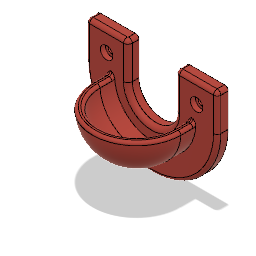
BallCatcher (Autodesk Fusion 360 design; units mm, degrees)
Autodesk Fusion 360 part; units mm, degrees
sphere "SpherePrimitive1" add diameter 60 placed x (1, 0, 0) y (0, 0, -1) z (0, 1, 0) at (0, 0, 0) makes body 1
shell "Shell1" thickness 5 removed faces 0 bodies 1
split "Split1" by plane through (0, 0, 0) normal (0, 0, 1) bodies 1 makes body 2 at (28.4422, -6.3836, 7.0914)
split "Split2" by plane through (0, 0, 0) normal (0, 1, 0) bodies 2 makes body 3 at (-14.8717, 3.9158, 25.7585)
extrude "Extrude1" add 1 faces at (-2.6091, -28.1467, 0) along direction (0, 0, -1) blind 10 on bodies 2 bodies 2
sketch "Sketch2" plane through (0, 0, -10) normal (0, 0, -1) x (-1, 0, 0)
  line L0 (-25, 0) -> (-30, 0)
  arc A0 (-30, 0) -> (30, 0) centre (0, 0) ccw
  line L1 (30, 0) -> (25, 0)
  arc A1 (-25, 0) -> (25, 0) centre (0, 0) ccw
  line L2 (-25, 0) -> (25, 0)
  line L3 (0, 0) -> (48, 0)
  line L4 (0, 0) -> (-53, 0)
  arc A2 (-10.5, 0) -> (10.5, 0) centre (0, 0) ccw
  arc A3 (25, 14.5) -> (10.5, 0) centre (25, 0) ccw
  line L5 (42.0714, 14.5) -> (25, 14.5)
  arc A4 (-42.0714, 14.5) -> (42.0714, 14.5) centre (0, 0) ccw
  line L6 (-25, 14.5) -> (-42.0714, 14.5)
  arc A5 (-10.5, 0) -> (-25, 14.5) centre (-25, 0) ccw
  circle A6 centre (0, 0) radius 16
  dimension "d6" = 14.5
  dimension "d11" = 32
  constraint coincident A0.centre A1.centre
  constraint parallel L2 L3
  constraint parallel L2 L4
  measures "d11" diameter of A6
extrude "Extrude2" add sketch "Sketch2" along normal blind 8 contours L0 A0 L1 A1 L3 L4 | A1 L2 L3 L4 A6 | A0 L3 L4 A4 bodies 2
fillet "Fillet1" radius 3 1 edges at (0, -16, -10) on bodies 2
sketch "Sketch4" plane through (0, 0, 0) normal (0, 1, 0) x (-1, 0, 0)
  arc A0 (19, -10) -> (16, -13) centre (19, -13) ccw
  line L0 (16, -13) -> (16, -18)
  line L1 (16, -18) -> (44.5, -18)
  line L2 (44.5, -18) -> (44.5, -10)
  line L3 (44.5, -10) -> (30, -10)
  line L4 (30, -10) -> (30, 0)
  arc A1 (30, 0) -> (-30, 0) centre (0, 0) ccw
  line L5 (-30, 0) -> (-30, -10)
  line L6 (-30, -10) -> (-44.5, -10)
  line L7 (-44.5, -10) -> (-44.5, -18)
  line L8 (-44.5, -18) -> (-16, -18)
  line L9 (-16, -18) -> (-16, -13)
  arc A2 (-16, -13) -> (-19, -10) centre (-19, -13) ccw
  line L10 (-19, -10) -> (-25, -10)
  line L11 (-25, -10) -> (-25, 0)
  arc A3 (25, 0) -> (-25, 0) centre (0, 0) ccw
  line L12 (25, 0) -> (25, -10)
  line L13 (25, -10) -> (19, -10)
  line L14 (30, -10) -> (25, -10)
  line L15 (-25, -10) -> (-30, -10)
  constraint coincident L3.end L4.start
  constraint coincident L12.end L13.start
  constraint coincident L10.end L11.start
  constraint coincident L5.end L6.start
extrude "Extrude3" add sketch "Sketch4" along normal blind 25 contours A0 L0 L1 L2 L3 L13 L14 | L6 L7 L8 L9 A2 L10 L15 bodies 2
fillet "Fillet2" radius 1.903 1 faces at (26.6667, 0, -6.6667) on bodies 2
fillet "Fillet5" radius 2.5 11 edges at (44.5, 12.5, -10) (0, -44.5, -10) (-44.5, 12.5, -10) (-44.5, 25, -14) (-31.75, 25, -10) (-16.8787, 25, -10.8787) (-16, 25, -15.5) (16, 25, -15.5) (16.8787, 25, -10.8787) (31.75, 25, -10) (44.5, 25, -14) on bodies 2
sketch "Sketch3" plane through (0, 0, -10) normal (0, 0, 1) x (1, 0, 0)
  line L0 (26.8356, 1.903) -> (28.0325, 1.903)
  arc A0 (-29.9631, -1.4874) -> (29.9631, -1.4874) centre (0, 0) ccw
  line L1 (0, -43) -> (0, -30)
  line L2 (0, 0) -> (43, 0) construction
  line L3 (0, 0) -> (43, 0) construction
  arc A1 (-24.9665, -1.2946) -> (24.9665, -1.2946) centre (0, 0) ccw
  spline S0 degree 3 poles (24.9665, -1.2946) (24.9803, -1.0285) (25.038, -0.6917) (25.5642, 0.5413) (26.222, 1.1928) (26.8322, 1.899) (26.8339, 1.901) (26.8356, 1.903) knots 0 0 0 0 0.079915 0.079915 0.246548 0.246548 0.247022 0.247022 0.247022 0.247022
  spline S1 degree 3 poles (28.0325, 1.903) (28.0347, 1.901) (28.037, 1.899) (28.4413, 1.5442) (28.8666, 1.144) (29.4212, 0.3929) (29.6707, 0) (29.9285, -0.8103) (29.9799, -1.1484) (29.9631, -1.4874) knots -0.000904 -0.000904 -0.000904 -0.000904 0 0 0.160455 0.160455 0.251665 0.251665 0.312705 0.312705 0.312705 0.312705
  spline S2 degree 3 poles (-29.9631, -1.4874) (-29.9799, -1.1484) (-29.9285, -0.8103) (-29.6707, 0) (-29.4212, 0.3929) (-28.8666, 1.144) (-28.4413, 1.5442) (-28.037, 1.899) (-28.0347, 1.901) (-28.0325, 1.903) knots 0 0 0 0 0.101851 0.101851 0.254043 0.254043 0.521775 0.521775 0.523283 0.523283 0.523283 0.523283
  line L4 (-28.0325, 1.903) -> (-26.8356, 1.903)
  spline S3 degree 3 poles (-26.8356, 1.903) (-26.8339, 1.901) (-26.8322, 1.899) (-26.222, 1.1928) (-25.5642, 0.5413) (-25.038, -0.6917) (-24.9803, -1.0285) (-24.9665, -1.2946) knots -0.000794 -0.000794 -0.000794 -0.000794 0 0 0.279172 0.279172 0.41306 0.41306 0.41306 0.41306
  line L5 (-19, 0) -> (-19, 22.5)
  line L6 (19, 22.5) -> (19, 0)
  arc A2 (-19, 0) -> (19, 0) centre (0, 0) ccw
  line L7 (-42.0005, -0.0495) -> (-19, 22.5)
  line L8 (19, 22.5) -> (42.0005, -0.0495)
  line L9 (-19, 22.5) -> (-42, 22.5)
  line L10 (-42, 22.5) -> (-42, 0)
  arc A3 (-42, 0) -> (42, 0) centre (0, 0) ccw
  line L11 (42, 0) -> (42, 22.5)
  line L12 (42, 22.5) -> (19, 22.5)
  point P0 (-30.5002, 11.2252)
  point P1 (30.5002, 11.2252)
  constraint midpoint A0 L1.end
  constraint horizontal L2
  constraint coincident A0.centre L2.start
  constraint horizontal L3
  constraint coincident L5.end L7.end
  constraint coincident L6.start L8.start
  constraint midpoint L7 P0
  constraint midpoint L8 P1
hole "Hole2" at (-30.5002, 11.2252, -10) at (30.5002, 11.2252, -10) direction (0, 0, -1) diameter 4.6 depth 10 tip angle 180 counterbore diameter 8.5 counterbore depth 3.4 bodies 2
chamfer "Chamfer2" distance 0.5 angle 45 14 edges at (16, 11.25, -18) (0, -16, -18) (-16, 11.25, -18) (-16.7322, 24.2678, -18) (-30.25, 25, -18) (-43.7678, 24.2678, -18) (-44.5, 11.25, -18) (0, -44.5, -18) (44.5, 11.25, -18) (43.7678, 24.2678, -18) (30.25, 25, -18) (16.7322, 24.2678, -18) (28.3559, 10.3935, -18) (-32.6446, 10.3935, -18) on bodies 2
hidden bodies 1 3
equation "d1 = 50 mm + 2 * 5 mm"
equation "d11 = 27 mm + 5 mm"
